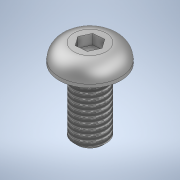
# Autodesk Inventor part: Tornillo allen cabeza boton M5
Saved by Autodesk Inventor 2020 (Build 240168000, 168)
## iProperties
Created: 2020-07-10
Part Number: Tornillo allen cabeza boton M5
Material: Genérico
Document SubType Name: Modeling
Designer: Pipi
Density: 1 g/cm^3
Appearance: Goma - Negro - Versión 1.1
Author: Pipi
Autodesk Inventor part; units mm, degrees
ref_plane "YZ Plane" through (0, 0, 0) normal (1, 0, 0) x (0, 1, 0)
ref_plane "XZ Plane" through (0, 0, 0) normal (0, 1, 0) x (-1, 0, 0)
ref_plane "XY Plane" through (0, 0, 0) normal (0, 0, 1) x (1, 0, 0)
sketch "Boceto1" plane through (0, 0, 0) normal (0, 1, 0) x (-1, 0, 0)
  circle A0 centre (0, 0) radius 2.5
  circle A1 centre (0, 0) radius 4.75
  dimension "d0" = 5
  dimension "d1" = 9.5
  constraints: 2 centre point, 2 coincident
  measures "d0" diameter of A0
  measures "d1" diameter of A1
extrude "Extrusión1" add sketch "Boceto1" along normal blind 2.75 contours A0 | A1
extrude "Extrusión2" add sketch "Boceto1" against normal blind 10 contours A0
thread "Rosca1" size "M5x0.8" class "6g" standard "ISO Metric profile" length 100
fillet "Empalme1" radius 2.25 1 edges at (4.75, 2.75, 0)
sketch "Boceto2" plane through (0, 2.75, 0) normal (0, 1, 0) x (1, 0, 0)
  line L0 (0.7249, 1.5731) -> (1.7248, 0.1588)
  line L1 (1.7248, 0.1588) -> (0.9999, -1.4143)
  line L2 (0.9999, -1.4143) -> (-0.7249, -1.5731)
  line L3 (-0.7249, -1.5731) -> (-1.7248, -0.1588)
  line L4 (-1.7248, -0.1588) -> (-0.9999, 1.4143)
  line L5 (-0.9999, 1.4143) -> (0.7249, 1.5731)
  point P0 (0, 0)
  point P1 (0, 0)
  dimension "d9" = 3
  constraints: 12 end point, 1 coincident, 13 other
  measures "d9" distance between parallel lines of L2 L5
extrude "Extrusión3" cut sketch "Boceto2" against normal blind 1.56
chamfer "Chaflán1" distance 0.5 angle 45 1 edges at (2.5, -10, 0)
